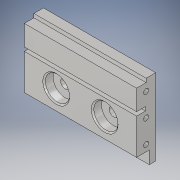
# Autodesk Inventor part: КВ33.000.102 - Стенка толстая
Saved by Autodesk Inventor 2019 (Build 230136000, 136)
## iProperties
Created: 2021-04-18
Part Number: КВ33.000.102 - Стенка толстая
Material: Steel
Document SubType Name: Modeling
Designer: Петров Иван
Density: 7.85 g/cm^3
Appearance: Aluminum - Dark
Author: Петров Иван
Autodesk Inventor part; units mm, degrees
ref_plane "YZ Plane" through (0, 0, 0) normal (1, 0, 0) x (0, 1, 0)
ref_plane "XZ Plane" through (0, 0, 0) normal (0, 1, 0) x (-1, 0, 0)
sketch "Sketch1" plane through (0, 0, 0) normal (0, 0, 1) x (1, 0, 0)
  line L0 (0, 0) -> (88, 0)
  line L1 (88, 0) -> (88, 10)
  line L2 (88, 10) -> (0, 10)
  line L3 (0, 10) -> (0, 0)
  dimension "d0" = 88
  dimension "d1" = 10
  constraints: 8 end point, 2 parallel, 1 horizontal, 1 perpendicular
  measures "d0" distance of L2.end L1.end
  measures "d1" distance of L1.end L0.end
extrude "Extrusion1" add sketch "Sketch1" along normal blind 5
sketch "Sketch2" plane through (0, 10, 0) normal (0, 1, 0) x (1, 0, 0)
  line L0 (0, 0) -> (88, 0)
  line L1 (88, 0) -> (88, -15)
  line L2 (88, -15) -> (0, -15)
  line L3 (0, -15) -> (0, 0)
  dimension "d4" = 88
  dimension "d5" = 15
  constraints: 8 end point, 2 parallel, 1 horizontal, 1 perpendicular
  measures "d4" distance of L1.end L2.end
  measures "d5" distance of L0.end L1.end
extrude "Extrusion2" add sketch "Sketch2" along normal blind 50
sketch "Sketch4" plane through (0, 0, 0) normal (0, 0, -1) x (-1, 0, 0)
  line L0 (0, 0) -> (-88, 0) projected
  line L1 (-88, 0) -> (-88, 10) projected
  line L2 (-88, 10) -> (0, 10) projected
  line L3 (0, 10) -> (0, 0) projected
  point P0 (-78, 5)
  dimension "d10" = 10
  dimension "d11" = 5
  measures "d10" distance from line of L1 point (-78, 5)
  measures "d11" distance from line of L0 point (-78, 5)
hole "Hole1" at (78, 5, 0) direction (0, 0, 1) diameter 4 depth 10 tip angle 120 countersink diameter 8 countersink angle 90
pattern_linear "Rectangular Pattern1" count 5 spacing 17 along (-1, 0, 0) of "Hole1"
sketch "Sketch5" plane through (88, 0, 5) normal (1, 0, 0) x (0, 0, -1)
  line L0 (0, 10) -> (-10, 10) projected
  line L1 (-10, 10) -> (-10, 60) projected
  point P0 (5, 0)
  point P1 (-2.5, 15)
  dimension "d22" = 5
  dimension "d23" = 7.5
  measures "d22" distance from line of L0 point (-2.5, 15)
  measures "d23" distance from line of L1 point (-2.5, 15)
hole "Hole2" at (88, 15, 7.5) direction (-1, 0, 0) diameter 4 depth 8 tip angle 120
thread "Thread1" size "M4x0.7" class "6H" standard "ANSI Metric M Profile" full length
pattern_linear "Rectangular Pattern2" count 3 spacing 18 along (0, 1, 0) of "Hole2"
ref_plane "Work Plane1" through (44, 60, 0) normal (1, 0, 0) x (0, 0, -1)
mirror "Mirror1" about plane through (44, 60, 0) normal (1, 0, 0) of "Hole2", "Rectangular Pattern2"
sketch "Sketch6" plane through (0, 10, 15) normal (0, 0, 1) x (1, 0, 0)
  circle A0 centre (25, 15) radius 9.5
  line L0 (0, 50) -> (88, 50) projected
  line L1 (0, -10) -> (88, -10) projected
  point P0 (44, 50)
  dimension "d36" = 19
  dimension "d47" = 19
  dimension "d48" = 25
  constraints: 1 centre point, 1 midpoint
  measures "d36" diameter of A0
  measures "d47" horizontal distance of point (44, 50) A0.centre
  measures "d48" distance from line of L1 A0.centre
extrude "Extrusion3" cut sketch "Sketch6" against normal blind 7
sketch "Sketch7" plane through (25, 25, 8) normal (0, 0, 1) x (1, 0, 0)
  circle A0 centre (0, 0) radius 9.5 projected
  circle A1 centre (0, 0) radius 3.5
  point P0 (-25, -25)
  dimension "d39" = 7
  constraints: 1 centre point, 1 coincident
  measures "d39" diameter of A1
extrude "Extrusion4" cut sketch "Sketch7" against normal blind 58.5 and the other way blind 29.25 contours A1
chamfer "Chamfer1" distance 1 angle 45 1 edges at (15.5, 25, 15)
mirror "Mirror2" about plane through (44, 60, 0) normal (1, 0, 0) of "Extrusion4", "Extrusion3", "Chamfer1"
sketch "Sketch8" plane through (0, 60, 0) normal (0, 1, 0) x (1, 0, 0)
  line L0 (88, 0) -> (0, 0) projected
  line L1 (0, 0) -> (0, -15) projected
  line L2 (0, -15) -> (88, -15) projected
  line L3 (88, -15) -> (88, 0) projected
  line L4 (0, -15) -> (88, -15)
  line L5 (88, -15) -> (88, -7.5)
  line L6 (88, -7.5) -> (0, -7.5)
  line L7 (0, -7.5) -> (0, -15)
  constraints: 8 end point, 2 parallel, 1 horizontal, 1 midpoint, 1 perpendicular
extrude "Extrusion5" cut sketch "Sketch8" against normal blind 3 contours L3 L2 L1 L6
sketch "Sketch9" plane through (0, 0, 0) normal (0, 0, -1) x (-1, 0, 0)
  circle A0 centre (-81, 55) radius 2 projected
  circle A1 centre (-44, 55) radius 2 projected
  circle A2 centre (-7, 55) radius 2 projected
  point P0 (0, 0)
hole "Hole3" at (81, 55, 0) at (44, 55, 0) at (7, 55, 0) direction (0, 0, 1) diameter 4 depth 6.5 tip angle 120
sketch "Sketch10" plane through (88, 0, 5) normal (1, 0, 0) x (0, 0, -1)
  line L0 (-2.5, 60) -> (-2.5, 57) projected
  line L1 (-2.5, 57) -> (-10, 57) projected
  line L2 (-10, 10) -> (-10, 57) projected
  line L3 (0, 10) -> (-10, 10) projected
  line L4 (0, 0) -> (0, 10) projected
  line L5 (5, 0) -> (0, 0) projected
  line L6 (5, 0) -> (5, 60) projected
  line L7 (-2.5, 60) -> (5, 60) projected
  circle A0 centre (-2.5, 15) radius 2 projected
  circle A1 centre (-2.5, 33) radius 2 projected
  circle A2 centre (-2.5, 51) radius 2 projected
  line L8 (-10, 41) -> (-3, 41)
  line L9 (-3, 41) -> (-3, 38)
  line L10 (-3, 38) -> (-10, 38)
  line L11 (-10, 38) -> (-10, 41)
  dimension "d58" = 7
  dimension "d59" = 3
  dimension "d60" = 28
  constraints: 8 end point, 2 parallel, 1 horizontal, 1 perpendicular, 1 point on line
  measures "d58" distance of L9.end L10.end
  measures "d59" distance of L8.end L9.end
  measures "d60" distance between parallel lines of L3 L10
extrude "Extrusion6" cut sketch "Sketch10" against normal blind 114.5 contours L8 L9 L10 L2
equation "\"d10\" = hole_l_offset"
equation "\"d11\" = hole_h_offset"
equation "\"d21\" = hole_step"
equation "\"hole_l_offset\" = 10"
equation "\"hole_step\" = 17"
equation "\"hole_h_offset\" = 5"
body "Solid1"
